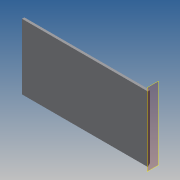
# Autodesk Inventor part: cover plate
Saved by Autodesk Inventor 2013 (Build 170138000, 138)
## iProperties
Created: 2017-04-06
Part Number: cover plate
Material: Generic
Document SubType Name: Modeling
Designer: employee
Density: 1 g/cm^3
Author: employee
Autodesk Inventor part; units mm, degrees
ref_plane "YZ Plane" through (0, 0, 0) normal (1, 0, 0) x (0, 1, 0)
ref_plane "XZ Plane" through (0, 0, 0) normal (0, 1, 0) x (-1, 0, 0)
ref_plane "XY Plane" through (0, 0, 0) normal (0, 0, 1) x (1, 0, 0)
ref_plane "Work Plane1" through (127.85, -14.5, 0) normal (-1, 0, 0) x (0, 0, 1)
sketch "Sketch1" plane through (127.85, -14.5, 0) normal (-1, 0, 0) x (0, 0, 1)
  line L0 (-8.6, -47) -> (-8.6, 0) projected
  line L1 (0, -55.6) -> (-8.6, -47) projected
  line L2 (0, 0) -> (0, -55.6) projected
  line L3 (0, 0) -> (-8.6, 0) projected
  line L4 (-2, -4) -> (-2, -38) projected
  line L5 (-2, -38) -> (-2, -53.2464)
  line L6 (-2, -53.2464) -> (0, -55.2464)
  line L7 (-2, -4) -> (-2, -0.25)
  line L8 (-2, -0.25) -> (0, -0.25)
  point P0 (0, 14.5)
  dimension "d0" = 0.25
  dimension "d1" = 0.25
  constraints: 8 end point, 2 point on line, 1 collinear, 1 parallel, 1 perpendicular, 1 vertical
  measures "d0" distance between parallel lines of L1 L6
  measures "d1" distance between parallel lines of L3 L8
extrude "Extrusion1" add sketch "Sketch1" along normal blind 105.7 contours L6 L5 L4 L7 L8 L2
sketch "Sketch2" plane through (127.85, -69.7464, 0) normal (0, 0, 1) x (1, 0, 0)
  circle A0 centre (-21.25, 31.7464) radius 16 projected
  line L0 (-95.4365, 49.7602) -> (-42.9635, 49.7602) projected
  line L1 (-95.4365, 18.7327) -> (-95.4365, 49.7602) projected
  line L2 (-42.9635, 18.7327) -> (-95.4365, 18.7327) projected
  line L3 (-42.9635, 49.7602) -> (-42.9635, 18.7327) projected
  circle A1 centre (-21.25, 31.7464) radius 17
  point P0 (-127.85, 69.7464)
  dimension "d4" = 1
  constraints: 1 centre point
  measures "d4" radial gap between concentric circles of A0 A1
extrude "Extrusion2" cut sketch "Sketch2" against normal through all contours A0 | L0 L3 L2 L1 | A1
chamfer "Chamfer1" distance 2 angle 45 4 edges at (58.65, -19.9862, 0) (32.4135, -35.5, 0) (58.65, -51.0138, 0) (84.8865, -35.5, 0)
sketch "Sketch3" plane through (127.85, -69.7464, 0) normal (0, 0, 1) x (1, 0, 0)
  circle A0 centre (-6.75, 51.2464) radius 1.75 projected
  circle A1 centre (-101.7, 21.6214) radius 1.75 projected
  circle A2 centre (-101.7, 41.8714) radius 1.75 projected
  circle A3 centre (-6.75, 12.2464) radius 1.75 projected
  line L0 (-97.95, 25.9964) -> (-105.45, 25.9964) projected
  line L1 (-105.45, 25.9964) -> (-105.45, 8.7464) projected
  line L2 (-105.45, 8.7464) -> (-0.25, 8.7464) projected
  line L3 (-0.25, 8.7464) -> (-0.25, 54.7464) projected
  line L4 (-0.25, 54.7464) -> (-105.45, 54.7464) projected
  line L5 (-105.45, 54.7464) -> (-105.45, 37.4964) projected
  line L6 (-105.45, 37.4964) -> (-97.95, 37.4964) projected
  line L7 (-97.95, 37.4964) -> (-97.95, 51.2464) projected
  line L8 (-97.95, 51.2464) -> (-40.45, 51.2464) projected
  line L9 (-40.45, 51.2464) -> (-40.45, 17.2464) projected
  line L10 (-40.45, 17.2464) -> (-97.95, 17.2464) projected
  line L11 (-97.95, 17.2464) -> (-97.95, 25.9964) projected
  circle A4 centre (-21.25, 31.7464) radius 16 projected
  point P0 (-127.85, 69.7464)
extrude "Extrusion3" cut sketch "Sketch3" against normal through all contours A0 | A1 | A2 | A3
sketch "Sketch4" plane through (127.85, -67.7464, -2) normal (0, 0, -1) x (-1, 0, 0)
  circle A0 centre (101.7, 39.8714) radius 1.75 projected
  circle A1 centre (6.75, 49.2464) radius 1.75 projected
  circle A2 centre (101.7, 19.6214) radius 1.75 projected
  circle A3 centre (6.75, 10.2464) radius 1.75 projected
  circle A4 centre (6.75, 49.2464) radius 3
  circle A5 centre (6.75, 10.2464) radius 3
  circle A6 centre (101.7, 39.8714) radius 3
  circle A7 centre (101.7, 19.6214) radius 3
  point P0 (127.85, 67.7464)
  dimension "d12" = 6
  constraints: 4 centre point, 3 equal radius, 2 coincident
  measures "d12" diameter of A5
ref_plane "Work Plane2" through (22.4, -61, -7) normal (0, 0, 1) x (1, 0, 0)
extrude "Extrusion4" add sketch "Sketch4" along normal up to surface (5 mm away)
sketch "Sketch5" plane through (127.85, -67.7464, -2) normal (0, 0, -1) x (-1, 0, 0)
  line L0 (0, 0) -> (105.7, 0) projected
  line L1 (0, 52.9964) -> (105.7, 52.9964) projected
  line L2 (95.4365, 52.9964) -> (99.95, 52.9964)
  line L3 (99.95, 52.9964) -> (99.95, 0)
  line L4 (99.95, 0) -> (95.4365, 0)
  line L5 (95.4365, 0) -> (95.4365, 52.9964)
  circle A0 centre (101.7, 39.8714) radius 1.75 projected
  point P0 (95.4365, 47.7602)
  point P1 (127.85, 67.7464)
  constraints: 8 end point, 3 point on line, 2 parallel, 1 horizontal, 1 perpendicular, 1 tangent
extrude "Extrusion5" cut sketch "Sketch5" along normal through all contours L5 L1 L3 L0
sketch "Sketch6" plane through (127.85, -69.7464, 0) normal (0, 0, 1) x (1, 0, 0)
  circle A0 centre (-101.7, 41.8714) radius 1.75 projected
  circle A1 centre (-6.75, 51.2464) radius 1.75 projected
  circle A2 centre (-101.7, 21.6214) radius 1.75 projected
  circle A3 centre (-6.75, 12.2464) radius 1.75 projected
  point P0 (-127.85, 69.7464)
extrude "Extrusion6" add sketch "Sketch6" against normal blind 0.5
sketch "Sketch7" plane through (26.15, -48.125, -7) normal (0, 0, -1) x (-1, 0, 0)
  line L0 (-1.75, 2.4367) -> (-1.75, 0) projected
  circle A0 centre (0, 0) radius 1.75 projected
  line L1 (-1.75, 0) -> (-1.75, -2.4367) projected
  arc A1 (-1.75, -2.4367) -> (-1.75, 2.4367) centre (0, 0) ccw projected
  circle A2 centre (0, 20.25) radius 1.75 projected
  circle A3 centre (-94.95, 29.625) radius 1.75 projected
  circle A4 centre (-94.95, -9.375) radius 1.75 projected
  circle A5 centre (-94.95, 29.625) radius 1.5
  circle A6 centre (-94.95, -9.375) radius 1.5
  circle A7 centre (0, 0) radius 1.5
  circle A8 centre (0, 20.25) radius 1.5
  point P0 (26.15, 48.125)
  dimension "d20" = 3
  constraints: 4 centre point, 3 equal radius, 1 horizontal alignment
  measures "d20" diameter of A8
extrude "Extrusion7" add sketch "Sketch7" against normal up to surface (7 mm away) contours A0 | A1 L1 L0 | A2 | A3 | A4
sketch "Sketch8" plane through (26.15, -27.875, -7) normal (0, 0, -1) x (-1, 0, 0)
  line L0 (-1.75, 2.4367) -> (-1.75, -2.4367) projected
  arc A0 (-1.75, -2.4367) -> (-1.75, 2.4367) centre (0, 0) ccw projected
  arc A1 (-2.55, -1.5803) -> (-1.75, -2.4367) centre (0, 0) ccw
  line L1 (-2.55, -1.5803) -> (-2.55, 1.5803)
  arc A2 (-1.75, 2.4367) -> (-2.55, 1.5803) centre (0, 0) ccw
  arc A3 (-1.75, -22.6867) -> (-1.75, -17.8133) centre (0, -20.25) ccw projected
  arc A4 (-2.55, -21.8303) -> (-2.55, -18.6697) centre (0, -20.25) ccw
  line L2 (-2.55, -18.6697) -> (-2.55, -21.8303)
  line L3 (-1.75, -17.8133) -> (-1.75, -22.6867) projected
  point P0 (26.15, 27.875)
  dimension "d24" = 0.8
  dimension "d25" = 0.8
  constraints: 6 point on circle, 5 concentric, 4 end point, 3 centre point, 1 coincident, 1 collinear, 1 parallel
  measures "d24" distance between parallel lines of L1 L0
  measures "d25" distance between parallel lines of L3 L2
extrude "Extrusion8" add sketch "Sketch8" against normal up to surface (7 mm away) contours L0 A1 L1 A2 | A4 L2 L3
body "Solid1"
